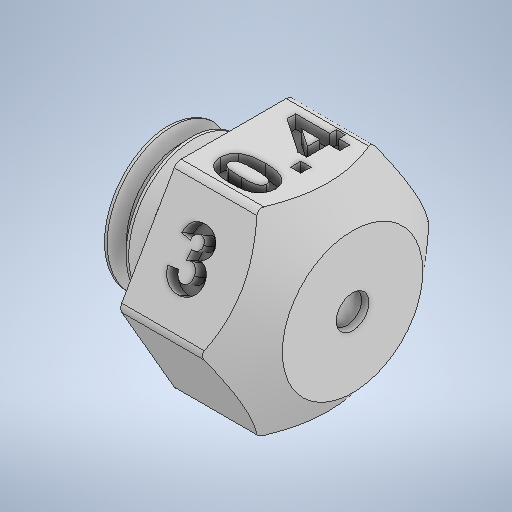
# Autodesk Inventor part: Part1
Saved by Autodesk Inventor 2025.2 (Build 292293000, 293)
## iProperties
Created: 2026-03-09
Part Number: Part1
Material: Generic
Document SubType Name: Modeling
Designer: Simon
Density: 1 g/cm^3
Appearance: Default
Author: Simon
Autodesk Inventor part; units mm, degrees
ref_plane "YZ Plane" through (0, 0, 0) normal (1, 0, 0) x (0, 1, 0)
ref_plane "XZ Plane" through (0, 0, 0) normal (0, 1, 0) x (-1, 0, 0)
ref_plane "XY Plane" through (0, 0, 0) normal (0, 0, 1) x (1, 0, 0)
sketch "Sketch1" plane through (0, 0, 0) normal (0, 0, 1) x (1, 0, 0)
  line L0 (0, 0) -> (0, 1.25)
  line L1 (0, 1.25) -> (50, 1.25)
  line L2 (0, 0) -> (0, 0.5544)
  line L3 (0, 0.5544) -> (50, 0.5544)
  line L4 (0, 0) -> (0, 0.6122)
  line L5 (0, 0.6122) -> (50, 0.6122)
  line L6 (0, 0) -> (0, 2.5)
  line L7 (0, 2.5) -> (2.5, 2.5)
  line L8 (2.5, 2.5) -> (2.5, 1.25)
  line L9 (2.5, 1.25) -> (2.5, 4.25)
  line L10 (2.5, 1.25) -> (6.7109, 1.25) construction
  line L11 (2.5, 4.25) -> (5.5, 4.25)
  line L12 (5.5, 4.25) -> (5.5, 1.25)
  line L13 (5.5, 1.25) -> (6.7048, 0.5544)
  line L14 (5.5, 1.25) -> (9.25, 1.25) construction
  line L15 (6.7048, 0.5544) -> (6.9207, 0.6122)
  line L16 (6.7048, 0.5544) -> (6.9284, 0.5544) construction
  line L17 (6.9207, 0.6122) -> (6.9207, 2.6122)
  line L18 (6.9207, 2.6122) -> (5.5, 4.25)
  line L19 (0, 0) -> (50, 0)
  dimension "d0" = 1.25
  dimension "d1" = 50
  dimension "d2" = 0.5544
  dimension "d3" = 0.6122
  dimension "d4" = 2.5
  dimension "d5" = 2.5
  dimension "d6" = 3
  dimension "d8" = 3
  dimension "d9" = 30
  dimension "d10" = 15
  dimension "d12" = 2
  dimension "d13" = 50
  constraints: 40 end point, 7 perpendicular, 7 point on line, 5 horizontal, 2 vertical, 1 equal length
  measures "d0" distance of L0.start L0.end
  measures "d1" distance of L0.end L1.end
  measures "d2" distance of L0.start L2.end
  measures "d3" distance of L0.start L4.end
  measures "d4" distance of L0.start L6.end
  measures "d5" distance of L6.end L7.end
  measures "d6" distance of L8.end L9.end
  measures "d8" distance of L9.end L11.end
  measures "d9" angle of L13 L14
  measures "d10" angle of L16 L15
  measures "d12" distance of L15.end L17.end
  measures "d13" distance of L0.start L19.end
revolve "Revolution1" add sketch "Sketch1" angle 360 about axis through (0, 0, 0) along (1, 0, 0) contours L13 L5 L15 | L6 L7 L8 L1 | L13 L1 L17 L5 | L8 L9 L11 L12 L1 | L12 L18 L17 L1
sketch "Sketch2" plane through (2.5, 0, 0) normal (-1, 0, 0) x (0, 0, 1)
  circle A0 centre (0, 0) radius 4.25 projected
  line L0 (-4.25, 0) -> (4.25, 0)
  circle A1 centre (0, 0) radius 0.5544 projected
  line L1 (4.25, 0) -> (2.125, -3.6806)
  line L2 (2.125, -3.6806) -> (-2.125, -3.6806)
  line L3 (-2.125, -3.6806) -> (-4.25, 0)
  line L4 (-4.25, 0) -> (-2.125, 3.6806)
  line L5 (-2.125, 3.6806) -> (2.125, 3.6806)
  line L6 (2.125, 3.6806) -> (4.25, 0)
  circle A2 centre (0, 0) radius 1.25
  constraints: 14 end point, 2 coincident, 2 point on circle, 1 centre point, 1 horizontal, 13 other
extrude "Extrusion1" cut sketch "Sketch2" against normal through all contours L6 A0 | A0 L1 | L5 A0 | A0 L2 | L4 A0 | A0 L3
fillet "Fillet1" radius 0.3 6 edges at (4, 3.6806, 2.125) (4, 3.6806, -2.125) (4, 0, -4.25) (4, -3.6806, -2.125) (4, -3.6806, 2.125) (4, 0, 4.25)
sketch "Sketch3" plane through (0, 0, 0) normal (0, 0, 1) x (1, 0, 0)
  line L0 (-0.35, 1.8938) -> (0.45, 1.8938)
  line L1 (-0.35, 1.8938) -> (0.05, 2.5866)
  line L2 (-0.35, 1.8938) -> (0.45, 1.8938) construction
  line L3 (0.05, 2.5866) -> (0.45, 1.8938)
  line L4 (-0.0972, 3.8266) -> (0.7028, 3.8266) construction
  line L5 (0.05, 2.5866) -> (0.05, 1.8938)
  line L6 (0.05, 1.8938) -> (0.05, 2.0671)
  line L7 (0.05, 2.0671) -> (0.45, 2.0671)
  line L8 (0.45, 2.0671) -> (-0.35, 2.0671)
  line L9 (0.05, 2.5866) -> (0.05, 2.5)
  line L10 (0.05, 2.5) -> (0.45, 2.5)
  line L11 (0.45, 2.5) -> (-0.35, 2.5)
  line L12 (-0.35, 1.8938) -> (-1.15, 1.8938)
  line L13 (0.05, 2.5866) -> (-0.75, 2.5866)
  line L14 (-0.75, 2.5866) -> (-1.15, 1.8938)
  line L15 (-0.35, 1.8938) -> (-0.75, 2.5866)
  line L16 (-0.35, 2.0671) -> (-1.15, 2.0671)
  line L17 (-0.35, 2.5) -> (-0.8, 2.5)
  line L18 (-0.75, 2.5866) -> (-0.75, 1.8938)
  line L19 (-0.35, 1.8938) -> (-0.35, 1.9938)
  circle A0 centre (-0.35, 2.0938) radius 0.1
  line L20 (-0.4077, 1.9938) -> (-0.2923, 1.9938)
  line L21 (0, 2.5) -> (2.5, 2.5) projected
  line L22 (0, 2.5) -> (-0.7, 2.5)
  line L23 (-0.7, 2.5) -> (-0.4366, 2.0438)
  line L24 (-0.4366, 2.0438) -> (-0.2634, 2.0438)
  line L25 (-0.2634, 2.0438) -> (0, 2.5)
  circle A1 centre (-0.35, 2.0938) radius 0.1
  point P0 (0, 0)
  point P1 (0, 2.5)
  dimension "d18" = 0.8
  dimension "d19" = 60
  dimension "d20" = 60
  dimension "d21" = 0.1732
  dimension "d22" = 0.0866
  dimension "d23" = 0.8
  dimension "d24" = 0.1
  dimension "d25" = 0.8
  constraints: 50 end point, 13 point on line, 7 horizontal, 4 tangent, 3 midpoint, 2 centre point, 2 equal length, 2 perpendicular, 2 point on circle, 1 coincident, 1 collinear, 1 concentric, 1 parallel, 1 vertical
  measures "d18" distance of L2.start L0.end
  measures "d19" angle of L2 L1
  measures "d20" angle of L3 L4
  measures "d21" distance of L6.start L7.start
  measures "d22" distance of L3.start L10.start
  measures "d23" distance of L2.start L12.end
  measures "d24" distance of L2.start L19.end
  measures "d25" distance between parallel lines of L5 L18
coil "Coil1" sketch "Sketch3" operation cut axis through (-10, 0, 0) along (1, 0, 0) pitch 0.8 turns 4 hand right contours A0 L24 | L24 L15 L16 L8 L1 | A0 L15 L17 L11 L1 | L8 L16 A0
extrude "Extrusion2" add sketch "Sketch2" against normal blind 3 contours L1 L2 L3 L0 A2 | L0 A2 L4 L5 L6
fillet "Fillet2" radius 0.3 6 edges at (4, 3.6806, -2.125) (4, 3.6806, 2.125) (4, 0, 4.25) (4, -3.6806, 2.125) (4, -3.6806, -2.125) (4, 0, -4.25)
sketch "Sketch4" plane through (2.5, 3.6806, 1.9518) normal (0, 1, 0) x (1, 0, 0)
  line L0 (0.6661, 0.0194) -> (0.6661, 3.902) construction
  line L1 (0.6661, 3.902) -> (2.7072, 3.902) construction
  line L2 (2.7072, 3.902) -> (2.7072, 0.0194) construction
  line L3 (2.7072, 0.0194) -> (0.6661, 0.0194) construction
  spline S0 degree 2 poles (0.6661, 0.7861) (0.6661, 1.0773) (0.8734, 1.2404) knots 0 0 0 1 1 1
  spline S1 degree 2 poles (0.8734, 1.2404) (1.1188, 1.4355) (1.6874, 1.4355) knots 0 0 0 1 1 1
  spline S2 degree 2 poles (1.6874, 1.4355) (2.2545, 1.4355) (2.503, 1.2389) knots 0 0 0 1 1 1
  spline S3 degree 2 poles (2.503, 1.2389) (2.7072, 1.0773) (2.7072, 0.7861) knots 0 0 0 1 1 1
  spline S4 degree 2 poles (2.7072, 0.7861) (2.7072, 0.4934) (2.2591, 0.1367) (1.6828, 0.1367) knots 0 0 0 1 2 2 2
  spline S5 degree 2 poles (1.6828, 0.1367) (1.1188, 0.1367) (0.8703, 0.3334) knots 0 0 0 1 1 1
  spline S6 degree 2 poles (0.8703, 0.3334) (0.6661, 0.495) (0.6661, 0.7861) knots 0 0 0 1 1 1
  spline S7 degree 2 poles (0.9847, 0.7861) (0.9847, 0.716) (1.0731, 0.6078) (1.1874, 0.5773) knots 0 0 0 1 2 2 2
  spline S8 degree 2 poles (1.1874, 0.5773) (1.3353, 0.5377) (1.6874, 0.5377) knots 0 0 0 1 1 1
  spline S9 degree 2 poles (1.6874, 0.5377) (2.038, 0.5377) (2.3017, 0.6093) (2.3886, 0.716) (2.3886, 0.7861) knots 0 0 0 1 2 3 3 3
  spline S10 degree 2 poles (2.3886, 0.7861) (2.3886, 0.8562) (2.3002, 0.9645) (2.1859, 0.995) knots 0 0 0 1 2 2 2
  spline S11 degree 2 poles (2.1859, 0.995) (2.038, 1.0346) (1.6874, 1.0346) knots 0 0 0 1 1 1
  spline S12 degree 2 poles (1.6874, 1.0346) (1.3353, 1.0346) (1.0731, 0.963) (0.9847, 0.8562) (0.9847, 0.7861) knots 0 0 0 1 2 3 3 3
  line L4 (2.6737, 1.7724) -> (2.2895, 1.7724)
  line L5 (2.2895, 1.7724) -> (2.2895, 2.1566)
  line L6 (2.2895, 2.1566) -> (2.6737, 2.1566)
  line L7 (2.6737, 2.1566) -> (2.6737, 1.7724)
  line L8 (2.6737, 3.2191) -> (2.2713, 3.2191)
  line L9 (2.2713, 3.2191) -> (2.2713, 2.4005)
  line L10 (2.2713, 2.4005) -> (1.9374, 2.4005)
  line L11 (1.9374, 2.4005) -> (0.6661, 3.2678)
  line L12 (0.6661, 3.2678) -> (0.6661, 3.5895)
  line L13 (0.6661, 3.5895) -> (1.9359, 3.5895)
  line L14 (1.9359, 3.5895) -> (1.9359, 3.838)
  line L15 (1.9359, 3.838) -> (2.2713, 3.838)
  line L16 (2.2713, 3.838) -> (2.2713, 3.5895)
  line L17 (2.2713, 3.5895) -> (2.6737, 3.5895)
  line L18 (2.6737, 3.5895) -> (2.6737, 3.2191)
  line L19 (1.9359, 3.2191) -> (1.2514, 3.2191)
  line L20 (1.2514, 3.2191) -> (1.9359, 2.7587)
  line L21 (1.9359, 2.7587) -> (1.9359, 3.2191)
  point P0 (-2.5, 1.9518)
  constraints: 2 other
extrude "Extrusion3" cut sketch "Sketch4" against normal blind 0.5
sketch "Sketch5" plane through (2.5, 0.15, 4.1634) normal (0, 0.5, 0.866) x (1, 0, 0)
  line L0 (0.8514, 3.0008) -> (2.4048, 3.0008) construction
  line L1 (2.4048, 3.0008) -> (2.4048, 0.9932) construction
  line L2 (2.4048, 0.9932) -> (0.8514, 0.9932) construction
  line L3 (0.8514, 0.9932) -> (0.8514, 3.0008) construction
  line L4 (0.9566, 1.5252) -> (1.3271, 1.5709)
  spline S0 degree 2 poles (1.3271, 1.5709) (1.3453, 1.4292) (1.5008, 1.2783) (1.6106, 1.2783) knots 0 0 0 1 2 2 2
  spline S1 degree 2 poles (1.6106, 1.2783) (1.7295, 1.2783) (1.8911, 1.4581) (1.8911, 1.6106) knots 0 0 0 1 2 2 2
  spline S2 degree 2 poles (1.8911, 1.6106) (1.8911, 1.7554) (1.7371, 1.9246) (1.6258, 1.9246) knots 0 0 0 1 2 2 2
  spline S3 degree 2 poles (1.6258, 1.9246) (1.5527, 1.9246) (1.4505, 1.8956) knots 0 0 0 1 1 1
  line L5 (1.4505, 1.8956) -> (1.4932, 2.2081)
  spline S4 degree 2 poles (1.4932, 2.2081) (1.6487, 2.2036) (1.8118, 2.3469) (1.8118, 2.4658) knots 0 0 0 1 2 2 2
  spline S5 degree 2 poles (1.8118, 2.4658) (1.8118, 2.5664) (1.6914, 2.6853) (1.5923, 2.6853) knots 0 0 0 1 2 2 2
  spline S6 degree 2 poles (1.5923, 2.6853) (1.4932, 2.6853) (1.3545, 2.5496) (1.3392, 2.4185) knots 0 0 0 1 2 2 2
  line L6 (1.3392, 2.4185) -> (0.9856, 2.478)
  spline S7 degree 2 poles (0.9856, 2.478) (1.0222, 2.6594) (1.1716, 2.8774) (1.4368, 3.0008) (1.603, 3.0008) knots 0 0 0 1 2 3 3 3
  spline S8 degree 2 poles (1.603, 3.0008) (1.885, 3.0008) (2.0557, 2.8209) knots 0 0 0 1 1 1
  spline S9 degree 2 poles (2.0557, 2.8209) (2.196, 2.6746) (2.196, 2.4886) knots 0 0 0 1 1 1
  spline S10 degree 2 poles (2.196, 2.4886) (2.196, 2.2264) (1.9078, 2.0694) knots 0 0 0 1 1 1
  spline S11 degree 2 poles (1.9078, 2.0694) (2.0801, 2.0328) (2.2844, 1.7752) (2.2844, 1.5938) knots 0 0 0 1 2 2 2
  spline S12 degree 2 poles (2.2844, 1.5938) (2.2844, 1.3301) (1.9002, 0.9597) (1.6136, 0.9597) knots 0 0 0 1 2 2 2
  spline S13 degree 2 poles (1.6136, 0.9597) (1.3423, 0.9597) (0.9856, 1.2722) (0.9566, 1.5252) knots 0 0 0 1 2 2 2
  point P0 (-2.5, 1.9518)
  constraints: 2 other
extrude "Extrusion4" cut sketch "Sketch5" against normal blind 0.5
body "Solid1"
